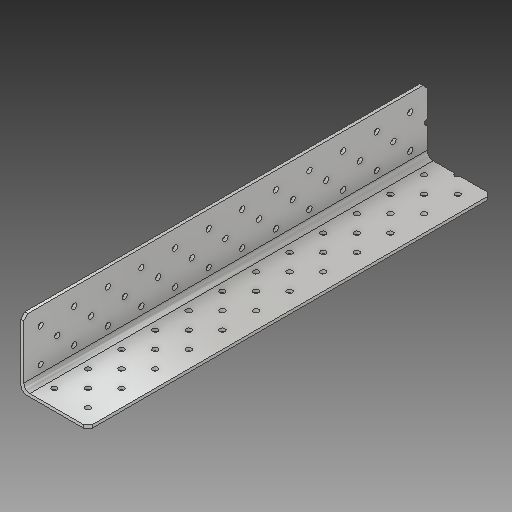
# Autodesk Inventor part: versaframe_angle-2x2
Saved by Autodesk Inventor 2017 (Build 210142000, 142)
## iProperties
Created: 2016-07-01
Part Number: versaframe_angle-2x2
Material: Aluminum 5052-H36
Document SubType Name: Modeling
Designer: rickab1
Density: 2.68277 g/cm^3
Appearance: Aluminum - Polished
Author: rickab1
Autodesk Inventor part; units mm, degrees
ref_plane "YZ Plane" through (0, 0, 0) normal (1, 0, 0) x (0, 1, 0)
ref_plane "XZ Plane" through (0, 0, 0) normal (0, 1, 0) x (-1, 0, 0)
ref_plane "XY Plane" through (0, 0, 0) normal (0, 0, 1) x (1, 0, 0)
sketch "Sketch1" plane through (0, 0, 0) normal (0, 0, 1) x (1, 0, 0)
  line L0 (0, 50.8) -> (0, 0)
  line L1 (0, 0) -> (50.8, 0)
  line L2 (50.8, 0) -> (50.8, 2.286)
  line L3 (50.8, 2.286) -> (2.286, 2.286)
  line L4 (2.286, 2.286) -> (2.286, 50.8)
  line L5 (2.286, 50.8) -> (0, 50.8)
  dimension "leg" = 50.8
  dimension "d1" = 2.286
  constraints: 12 end point, 7 perpendicular, 1 vertical
  measures "leg" distance of L0.start L0.end
  measures "d1" distance of L1.end L2.end
extrude "Extrusion1" add sketch "Sketch1" against normal blind 304.8
sketch "Sketch2" plane through (0, 0, 0) normal (-1, 0, 0) x (0, 0, 1)
  line L0 (0, 0) -> (0, 50.8) projected
  line L1 (0, 50.8) -> (-304.8, 50.8) projected
  line L2 (-304.8, 0) -> (-304.8, 50.8) projected
  line L3 (0, 0) -> (-304.8, 0) projected
  point P0 (-25.4, 25.4)
  dimension "d4" = 50.8
  dimension "d5" = 25.4
  dimension "hole_pos" = 25.4
  measures "d4" distance of L0.start L0.end
  measures "d5" distance from line of point (-25.4, 25.4) L3
  measures "hole_pos" distance from line of L0 point (-25.4, 25.4)
hole "Hole1" at (0, 25.4, -25.4) direction (1, 0, 0) diameter 4.0894 end through all
sketch "Sketch3" plane through (0, 0, 0) normal (0, -1, 0) x (1, 0, 0)
  line L0 (50.8, 0) -> (0, 0) projected
  line L1 (0, 0) -> (0, -304.8) projected
  line L2 (50.8, -304.8) -> (0, -304.8) projected
  line L3 (50.8, 0) -> (50.8, -304.8) projected
  point P0 (25.4, -25.4)
  dimension "d14" = 50.8
  dimension "d15" = 25.4
  dimension "d16" = 25.4
  measures "d14" distance of L0.start L0.end
  measures "d15" distance from line of L0 point (25.4, -25.4)
  measures "d16" distance from line of L1 point (25.4, -25.4)
hole "Hole2" at (25.4, 0, -25.4) direction (0, 1, 0) diameter 4.0894 end through all
sketch "Sketch4" plane through (0, 0, 0) normal (-1, 0, 0) x (0, 0, 1)
  circle A0 centre (-25.4, 25.4) radius 2.0447 projected
  line L0 (0, 0) -> (0, 50.8) projected
  line L1 (0, 50.8) -> (-304.8, 50.8) projected
  line L2 (-304.8, 0) -> (-304.8, 50.8) projected
  line L3 (0, 0) -> (-304.8, 0) projected
  point P0 (-12.7, 38.1)
  point P1 (-12.7, 12.7)
  dimension "d24" = 12.7
  dimension "d25" = 12.7
  dimension "d26" = 12.7
  constraints: 1 vertical alignment
  measures "d24" distance from line of L0 point (-12.7, 38.1)
  measures "d25" distance from line of L1 point (-12.7, 38.1)
  measures "d26" distance from line of L3 point (-12.7, 12.7)
hole "Hole3" at (0, 38.1, -12.7) at (0, 12.7, -12.7) direction (1, 0, 0) diameter 4.0894 end through all
sketch "Sketch5" plane through (0, 0, 0) normal (0, -1, 0) x (1, 0, 0)
  circle A0 centre (25.4, -25.4) radius 2.0447 projected
  line L0 (50.8, 0) -> (0, 0) projected
  line L1 (0, 0) -> (0, -304.8) projected
  line L2 (50.8, -304.8) -> (0, -304.8) projected
  line L3 (50.8, 0) -> (50.8, -304.8) projected
  point P0 (12.7, -12.7)
  point P1 (38.1, -12.7)
  dimension "d34" = 12.7
  dimension "d35" = 12.7
  dimension "d36" = 12.7
  constraints: 1 horizontal alignment
  measures "d34" distance from line of L1 point (12.7, -12.7)
  measures "d35" distance from line of L0 point (12.7, -12.7)
  measures "d36" distance from line of L3 point (38.1, -12.7)
hole "Hole4" at (12.7, 0, -12.7) at (38.1, 0, -12.7) direction (0, 1, 0) diameter 4.0894 end through all
chamfer "Chamfer1" distance 3.175 angle 45 4 edges at (1.143, 50.8, 0) (50.8, 1.143, 0) (1.143, 50.8, -304.8) (50.8, 1.143, -304.8)
fillet "Fillet1" radius 4.572 2 edges at (0, 0, -152.4) (2.286, 2.286, -152.4)
pattern_linear "Rectangular Pattern1" count 13 spacing 25.4 along (0, 0, -1) of "Hole1", "Hole2"
pattern_linear "Rectangular Pattern2" count 13 spacing 25.4 along (0, 0, -1) of "Hole3", "Hole4"
equation "\"d5\" = 0.5 * d4"
equation "\"d15\" = hole_pos"
equation "\"d16\" = 0.5 * d14"
equation "\"d26\" = d25"
equation "\"d36\" = d34"
body "Solid1"
